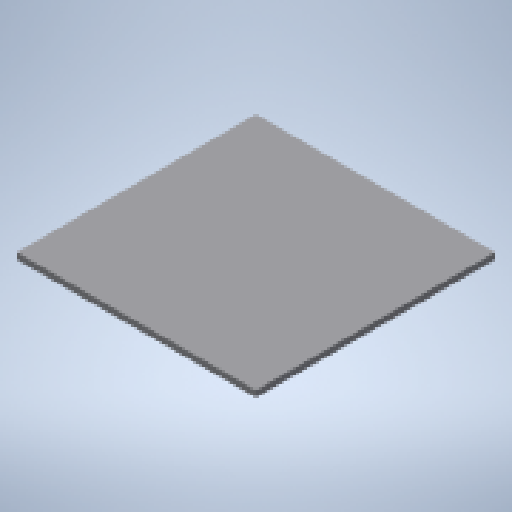
# Autodesk Inventor part: tabla40
Saved by Autodesk Inventor 2024 (Build 280153000, 153)
## iProperties
Created: 2024-04-03
Part Number: tabla40
Material: Generic
Document SubType Name: Modeling
Designer: compu
Density: 1 g/cm^3
Appearance: Default
Author: compu
Autodesk Inventor part; units mm, degrees
ref_plane "YZ Plane" through (0, 0, 0) normal (1, 0, 0) x (0, 1, 0)
ref_plane "XZ Plane" through (0, 0, 0) normal (0, 1, 0) x (-1, 0, 0)
ref_plane "XY Plane" through (0, 0, 0) normal (0, 0, 1) x (1, 0, 0)
sketch "Sketch1" plane through (0, 0, 0) normal (0, 1, 0) x (-1, 0, 0)
  line L0 (150, -150) -> (150, 150)
  line L1 (150, 150) -> (-150, 150)
  line L2 (-150, 150) -> (-150, -150)
  line L3 (-150, -150) -> (150, -150)
  line L4 (210, 0) -> (-210, 0) projected
  line L5 (0, -210) -> (0, 210) projected
  point P0 (0, 0)
  dimension "d0" = 300
  dimension "d1" = 300
  constraints: 8 end point, 2 perpendicular, 1 parallel, 1 vertical, 2 other
  measures "d0" distance of L0.start L0.end
  measures "d1" distance of L2.end L0.start
extrude "Extrusion1" add sketch "Sketch1" along normal blind 8
body "Solid1"
